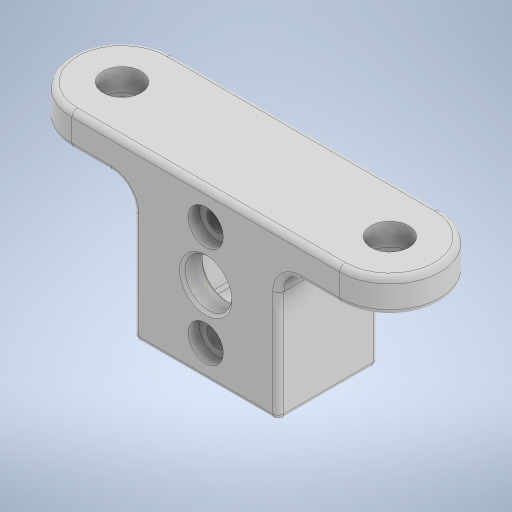
# Autodesk Inventor part: v2motormount
Saved by Autodesk Inventor 2024.2 (Build 282272000, 272)
## iProperties
Created: 2023-12-09
Part Number: v2motormount
Material: Generic
Document SubType Name: Modeling
Designer: Eric
Density: 1 g/cm^3
Appearance: Default
Author: Eric
Autodesk Inventor part; units mm, degrees
ref_plane "YZ Plane" through (0, 0, 0) normal (1, 0, 0) x (0, 1, 0)
ref_plane "XZ Plane" through (0, 0, 0) normal (0, 1, 0) x (-1, 0, 0)
ref_plane "XY Plane" through (0, 0, 0) normal (0, 0, 1) x (1, 0, 0)
sketch "Sketch1" plane through (0, 0, 0) normal (0, 1, 0) x (-1, 0, 0)
  point P0 (0, 0)
sketch "Sketch2" plane through (0, 0, 0) normal (0, 0, 1) x (1, 0, 0)
  circle A0 centre (0, -4.5) radius 0.9
  circle A1 centre (0, 4.5) radius 0.9
  circle A2 centre (0, 0) radius 2.0975
  line L0 (6.5, 7.5) -> (-6.5, 7.5)
  line L1 (-6.5, 7.5) -> (-6.5, -7.5)
  line L2 (-6.5, -7.5) -> (6.5, -7.5)
  line L3 (6.5, -7.5) -> (6.5, 7.5)
  dimension "d0" = 1.8
  dimension "d1" = 9
  dimension "d2" = 4.195
  dimension "d3" = 4.5
  dimension "d4" = 13
  dimension "d5" = 15
  dimension "d6" = 7.5
  dimension "d7" = 6.5
  constraints: 8 end point, 3 centre point, 2 parallel, 2 vertical alignment, 1 coincident, 1 equal radius, 1 horizontal, 1 perpendicular
  measures "d0" diameter of A1
  measures "d1" distance of A1.centre A0.centre
  measures "d2" diameter of A2
  measures "d3" distance of point (0, 0) A1.centre
  measures "d4" distance of L1.end L2.end
  measures "d5" distance of L2.end L0.start
  measures "d6" distance from line of point (0, 0) L0
  measures "d7" distance from line of point (0, 0) L3
extrude "Extrusion1" add sketch "Sketch2" against normal blind 2
sketch "Sketch3" plane through (0, 0, -2) normal (0, 0, -1) x (-1, 0, 0)
  line L0 (6.5, 7.5) -> (-6.5, 7.5) projected
  line L1 (-6.5, 7.5) -> (-6.5, -7.5) projected
  line L2 (6.5, -7.5) -> (6.5, 7.5) projected
  line L3 (-6.5, -7.5) -> (6.5, -7.5) projected
  line L4 (-5, 6) -> (5, 6)
  line L5 (5, 6) -> (5, -6)
  line L6 (5, -6) -> (-5, -6)
  line L7 (-5, -6) -> (-5, 6)
  point P0 (0, 0)
  dimension "d10" = 1.5
  dimension "d11" = 1.5
  dimension "d12" = 1.5
  dimension "d13" = 1.5
  constraints: 8 end point, 2 parallel, 1 horizontal, 1 perpendicular
  measures "d10" distance between parallel lines of L3 L6
  measures "d11" distance between parallel lines of L2 L5
  measures "d12" distance between parallel lines of L1 L7
  measures "d13" distance between parallel lines of L4 L0
extrude "Extrusion2" add sketch "Sketch3" along normal blind 7
sketch "Sketch4" plane through (-6.5, 7.5, 0) normal (0, 1, 0) x (1, 0, 0)
  line L0 (13, 9) -> (0, 9) projected
  line L1 (0, 9) -> (-10, 9)
  line L2 (-10, 9) -> (-10, 0)
  line L3 (0, 0) -> (13, 0) projected
  line L4 (-10, 0) -> (0, 0)
  line L5 (13, 0) -> (23, 0)
  line L6 (23, 0) -> (23, 9)
  line L7 (23, 9) -> (13, 9)
  line L8 (0, 0) -> (0, 9) projected
  line L9 (13, 0) -> (13, 9) projected
  circle A0 centre (-5.5, 4.5) radius 1.7
  circle A1 centre (18.5, 4.5) radius 1.7
  point P0 (6.5, 0)
  point P1 (-10, 4.5)
  point P2 (-5, 0)
  point P3 (18, 0)
  dimension "d16" = 3.4
  dimension "d17" = 10
  dimension "d22" = 4.5
  dimension "d23" = 4.5
  constraints: 12 end point, 3 midpoint, 3 perpendicular, 2 centre point, 2 collinear, 2 horizontal, 2 horizontal alignment, 1 equal radius
  measures "d16" diameter of A0
  measures "d17" distance between parallel lines of L8 L2
  measures "d22" distance from line of L2 A0.centre
  measures "d23" distance from line of L6 A1.centre
extrude "Extrusion3" add sketch "Sketch4" against normal blind 3 contours L7 L6 L5 L9 | L8 L4 L2 L1
fillet "Fillet1" radius 2 2 edges at (-6.5, 4.5, -4.5) (6.5, 4.5, -4.5)
fillet "Fillet2" radius 4.5 4 edges at (-16.5, 6, 0) (-16.5, 6, -9) (16.5, 6, 0) (16.5, 6, -9)
sketch "Sketch5" plane through (-6.5, 4.5, 0) normal (0, -1, 0) x (1, 0, 0)
  circle A0 centre (18.5, -4.5) radius 1.7 projected
  circle A1 centre (-5.5, -4.5) radius 1.7 projected
  circle A2 centre (18.5, -4.5) radius 2.625
  circle A3 centre (-5.5, -4.5) radius 2.625
  point P0 (6.5, 0)
  dimension "d24" = 5.25
  constraints: 2 centre point, 2 coincident, 1 equal radius
  measures "d24" diameter of A2
extrude "Extrusion4" cut sketch "Sketch5" against normal blind 1
fillet "Fillet3" radius 0.5 30 edges at (-6.5, -7.5, -4.5) (6.5, -7.5, -4.5) (-7.0858, 3.9142, 0) (-10.25, 4.5, 0) (-15.182, 4.5, -7.682) (-15.182, 4.5, -1.318) (-16.5, 4.5, -4.5) (-10.2501, 4.5, -9) (-7.0858, 3.9142, -9) (-6.5, -2.5, -9) (-6.5, -2.5, 0) (7.0858, 3.9142, 0) (10.25, 4.5, 0) (15.182, 4.5, -1.318) (16.5, 4.5, -4.5) (15.182, 4.5, -7.682) (10.25, 4.5, -9) (7.0858, 3.9142, -9) (6.5, -2.5, -9) (6.5, -2.5, 0) (0, -7.5, 0) (0, -7.5, -9) (0, 7.5, 0) (-16.5, 7.5, -4.5) (-15.182, 7.5, -7.682) (-15.182, 7.5, -1.318) (0, 7.5, -9) (15.182, 7.5, -7.682) (15.182, 7.5, -1.318) (16.5, 7.5, -4.5)
fillet "Fillet4" radius 0.25 4 edges at (5, -6, -5.5) (-5, -6, -5.5) (5, 6, -5.5) (-5, 6, -5.5)
chamfer "Chamfer1" distance 0.25 angle 45 10 edges at (-2.0975, 0, -2) (-2.0975, 0, 0) (0, -6, -9) (4.9268, -5.9268, -9) (5, 0, -9) (4.9268, 5.9268, -9) (0, 6, -9) (-4.9268, 5.9268, -9) (-5, 0, -9) (-4.9268, -5.9268, -9)
sketch "Sketch6" plane through (0, 0, 0) normal (0, 0, 1) x (1, 0, 0)
  circle A0 centre (0, 4.5) radius 0.9 projected
  circle A1 centre (0, 4.5) radius 1.575
  circle A2 centre (0, -4.5) radius 0.9 projected
  circle A3 centre (0, -4.5) radius 1.575
  point P0 (0, 0)
  dimension "d32" = 3.15
  constraints: 2 centre point, 2 coincident, 1 equal radius
  measures "d32" diameter of A1
extrude "Extrusion5" cut sketch "Sketch6" against normal blind 1
sketch "Sketch7" plane through (0, 4.5, -1) normal (0, 0, 1) x (1, 0, 0)
  circle A0 centre (0, 0) radius 0.9 projected
  circle A1 centre (0, -9) radius 0.9 projected
  point P0 (0, -4.5)
extrude "Extrusion6" [suppressed]
body "Solid1"
